Autodesk Fusion 360 part; units mm, degrees
note: some values were not read from the file. Set by a fixed rule: which face or edge a step refers to.
(part 5 of 5)
fillet "Fillet1''''''" radius 11.5 1 edges at (7, -47.65, -17.015) on bodies 23 in component "L_F_Wheel_Base"
fillet "Fillet2'''''''" radius 14 1 edges at (16, -47.65, -17.015) on bodies 23 in component "L_F_Wheel_Base"
sketch "Sketch5 (9)" plane through (0, 0, -26.015) normal (0, 0, -1) x (-1, 0, 0) in component "L_F_Wheel_Base"
  arc A0 (-16, -38.3973) -> (-10.1604, -49.7731) centre (-2, -38.3973) ccw
  arc A1 (-5.5, -57.351) -> (-10.1604, -49.7731) centre (-16.8635, -59.1175) ccw
  line L0 (-5.5, -57.351) -> (-5.5, -72.351)
  line L1 (-5.5, -72.351) -> (9.5, -72.351)
  line L2 (9.5, -72.351) -> (9.5, -57.351)
  line L3 (9.5, -57.351) -> (-7, -39.65)
  line L4 (-7, -39.65) -> (-7, -31.65)
  line L5 (-7, -31.65) -> (-16, -31.65)
  line L6 (-16, -31.65) -> (-16, -38.3973)
  line L7 (9.5, -57.351) -> (-5.5, -57.351)
  constraint coincident L2.end L3.start
  constraint coincident A1.start L0.start
extrude "Extrude5''''''''" add sketch "Sketch5 (9)" along normal blind 2 contours L0 L1 L2 L7 bodies 23 in component "L_F_Wheel_Base"
extrude "Extrude6''''''''" cut 1 faces at (0.5, -67.351, -6.015) along direction (0, 0, -1) blind 2 on bodies 23 bodies 23 in component "L_F_Wheel_Base"
sketch "Sketch6 (9)" plane through (0, -26.65, 0) normal (0, 1, 0) x (-1, 0, 0) in component "L_F_Wheel_Base"
  circle A0 centre (-11.5, -4.1) radius 1
  circle A1 centre (-11.5, -29.93) radius 1
  line L0 (-5.5, -29.015) -> (-5.5, -5.015)
  line L1 (-5.5, -5.015) -> (-7.1, -5.015)
  line L2 (-7.1, -5.015) -> (-7.1, -0.5642)
  line L3 (-7.1, -0.5642) -> (-15.9, -0.5642)
  line L4 (-15.9, -0.5642) -> (-15.9, -5.015)
  line L5 (-15.9, -5.015) -> (-17.5, -5.015)
  line L6 (-17.5, -5.015) -> (-17.5, -29.015)
  line L7 (-17.5, -29.015) -> (-15.9, -29.015)
  line L8 (-15.9, -29.015) -> (-15.9, -33.466)
  line L9 (-15.9, -33.466) -> (-7.1, -33.466)
  line L10 (-7.1, -33.466) -> (-7.1, -29.015)
  line L11 (-7.1, -29.015) -> (-5.5, -29.015)
  line L12 (-16, -27.03) -> (-7, -27.03)
  line L13 (-16, -7) -> (-16, -27.03)
  line L14 (-7, -27.03) -> (-7, -7)
  line L15 (-7, -27.03) -> (-16, -27.03)
  line L16 (-16, -27.03) -> (-16, -7)
  line L17 (-16, -7) -> (-7, -7)
  line L18 (-7, -7) -> (-7, -27.03)
  line L19 (-15.91, -7.09) -> (-7.09, -7.09)
  line L20 (-7.09, -7.09) -> (-7.09, -26.94)
  line L21 (-7.09, -26.94) -> (-15.91, -26.94)
  line L22 (-15.91, -26.94) -> (-15.91, -7.09)
  dimension "d553_1" = 0.09
  constraint horizontal L15
  constraint vertical L16
  constraint horizontal L17
  constraint vertical L18
  constraint coincident L13.start L16.end
  constraint coincident L12.end L14.start
extrude "Extrude7'''''" add sketch "Sketch6 (9)" along normal blind 3 contours L19 L20 L21 L22 bodies 23 in component "L_F_Wheel_Base"
sketch "Sketch7 (7)" plane through (0, 0, -8.015) normal (0, 0, 1) x (1, 0, 0) in component "L_F_Wheel_Base"
  arc A0 (10.1604, -49.7731) -> (16, -38.3973) centre (2, -38.3973) ccw
  line L0 (16, -38.3973) -> (16, -31.65)
  line L1 (16, -31.65) -> (7, -31.65)
  line L2 (7, -31.65) -> (7, -39.65)
  line L3 (7, -39.65) -> (-9.5, -57.351)
  line L4 (-9.5, -57.351) -> (-9.5, -72.351)
  line L5 (-9.5, -72.351) -> (5.5, -72.351)
  line L6 (5.5, -72.351) -> (5.5, -57.351)
  arc A1 (10.1604, -49.7731) -> (5.5, -57.351) centre (16.8635, -59.1175) ccw
  line L7 (-9.5, -57.351) -> (5.5, -57.351)
  circle A2 centre (-2, -64.851) radius 2
  line L8 (-2, -64.851) -> (-6.572, -64.851) construction
  line L9 (-2, -64.851) -> (2.572, -64.851) construction
  circle A3 centre (-6.572, -64.851) radius 0.75
  circle A4 centre (2.572, -64.851) radius 0.75
  dimension "d556_1" = 4
  dimension "d557_1" = 4.572
  dimension "d558_1" = 4.572
  dimension "d559_1" = 1.5
  dimension "d560_1" = 1.5
  constraint coincident L3.end L4.start
  constraint coincident L6.end A1.end
  constraint coincident A2.centre L8.start
  constraint horizontal L8
  constraint parallel L8 L9
  constraint coincident L8.end A3.centre
  constraint coincident L9.end A4.centre
  measures "d556_1" diameter of A2
  measures "d557_1" distance of A2.centre L8.end
  measures "d558_1" distance of A2.centre L9.end
  measures "d559_1" diameter of A3
  measures "d560_1" diameter of A4
extrude "Extrude8'''''" cut sketch "Sketch7 (7)" against normal blind 20 contours A2 | A3 | A4 bodies 23 in component "L_F_Wheel_Base"
sketch "Sketch8 (4)" plane through (0, 0, -28.015) normal (0, 0, -1) x (-1, 0, 0) in component "L_F_Wheel_Base"
  circle A0 centre (2, -64.851) radius 2
  circle A1 centre (6.572, -64.851) radius 0.75
  circle A2 centre (-2.572, -64.851) radius 0.75
  line L0 (9.5, -57.351) -> (-5.5, -57.351)
  line L1 (-5.5, -57.351) -> (-5.5, -72.351)
  line L2 (-5.5, -72.351) -> (9.5, -72.351)
  line L3 (9.5, -72.351) -> (9.5, -57.351)
  line L4 (8.1, -69.951) -> (-4.1, -69.951)
  line L5 (-4.1, -69.951) -> (-4.1, -59.751)
  line L6 (-4.1, -59.751) -> (8.1, -59.751)
  line L7 (8.1, -59.751) -> (8.1, -69.951)
  line L8 (8.1, -69.951) -> (-4.1, -59.751) construction
  line L9 (-4.1, -69.951) -> (8.1, -59.751) construction
  point P0 (2, -64.851)
  dimension "d563_1" = 12.2
  dimension "d564_1" = 10.2
  constraint horizontal L4
  constraint perpendicular L4 L5
  constraint parallel L4 L6
  constraint parallel L5 L7
  constraint coincident L8 P0
  constraint coincident L9 P0
  constraint coincident P0 A0.centre
  measures "d563_1" distance of L5.end L6.end
  measures "d564_1" distance of L4.end L5.end
extrude "Extrude9''''" cut sketch "Sketch8 (4)" against normal blind 18.841 contours L4 L5 L6 L7 bodies 23 in component "L_F_Wheel_Base"
extrude "Extrude10''" add 1 faces at (0.0333, -59.751, -21.7347) along direction (0, -1, 0) blind 10.2 on bodies 23 bodies 23 in component "L_F_Wheel_Base"
extrude "Extrude11''" cut 3 faces at (-1.7564, -64.1717, -9.174) (-6.3887, -65.021, -9.174) (2.2775, -64.681, -9.174) along direction (0, 0, -1) blind 18.841 on bodies 23 bodies 23 in component "L_F_Wheel_Base"
sketch "Sketch9 (2)" plane through (0, 0, -8.015) normal (0, 0, 1) x (1, 0, 0) in component "L_F_Wheel_Base"
  circle A0 centre (-2, -64.851) radius 2
  circle A1 centre (-6.572, -64.851) radius 0.75
  circle A2 centre (2.572, -64.851) radius 0.75
  arc A3 (10.1604, -49.7731) -> (16, -38.3973) centre (2, -38.3973) ccw
  line L0 (16, -38.3973) -> (16, -31.65)
  line L1 (16, -31.65) -> (7, -31.65)
  line L2 (7, -31.65) -> (7, -39.65)
  line L3 (7, -39.65) -> (-9.5, -57.351)
  line L4 (-9.5, -57.351) -> (-9.5, -72.351)
  line L5 (-9.5, -72.351) -> (5.5, -72.351)
  line L6 (5.5, -72.351) -> (5.5, -57.351)
  arc A4 (10.1604, -49.7731) -> (5.5, -57.351) centre (16.8635, -59.1175) ccw
  line L7 (-9.5, -57.351) -> (5.5, -57.351)
  constraint coincident L3.end L4.start
  constraint coincident L6.end A4.end
extrude "Extrude12''" add sketch "Sketch9 (2)" along normal blind 2 contours L4 L5 L6 L7 bodies 23 in component "L_F_Wheel_Base"
extrude "Extrude13'''" cut 1 faces at (-2.0498, -70.5158, -28.015) along direction (0, 0, 1) blind 2 on bodies 23 bodies 23 in component "L_F_Wheel_Base"
sketch "Sketch10 (2)" plane through (0, 0, -6.015) normal (0, 0, 1) x (1, 0, 0) in component "L_F_Wheel_Base"
  circle A0 centre (2.572, -64.851) radius 0.75
  circle A1 centre (-2, -64.851) radius 2
  circle A2 centre (-6.572, -64.851) radius 0.75
  line L0 (-9.5, -72.351) -> (5.5, -72.351)
  line L1 (5.5, -72.351) -> (5.5, -57.351)
  line L2 (5.5, -57.351) -> (-9.5, -57.351)
  line L3 (-9.5, -57.351) -> (-9.5, -72.351)
  line L4 (4.1, -69.951) -> (-8.1, -69.951)
  line L5 (-8.1, -69.951) -> (-8.1, -59.751)
  line L6 (-8.1, -59.751) -> (4.1, -59.751)
  line L7 (4.1, -59.751) -> (4.1, -69.951)
  line L8 (4.1, -69.951) -> (-8.1, -59.751) construction
  line L9 (-8.1, -69.951) -> (4.1, -59.751) construction
  point P0 (-2, -64.851)
  dimension "d575" = 12.2
  dimension "d576" = 10.2
  constraint horizontal L4
  constraint perpendicular L4 L5
  constraint parallel L4 L6
  constraint parallel L5 L7
  constraint coincident L8 P0
  constraint coincident L9 P0
  constraint coincident P0 A1.centre
  measures "d575" distance of L5.end L6.end
  measures "d576" distance of L4.end L5.end
extrude "Extrude14''" cut sketch "Sketch10 (2)" against normal blind 18.841 contours L4 L5 L6 L7 bodies 23 in component "L_F_Wheel_Base"
ref_plane "WorkPlane1" through (3.25, -52.0005, 1.985) normal (0, 0, 1) x (-1, 0, 0)
sketch "Sketch7 (1)" plane through (3.25, -52.0005, 1.985) normal (0, 0, 1) x (1, 0, 0)
  circle A0 centre (-5.25, -12.8505) radius 2
  circle A1 centre (-5.25, -12.8505) radius 25
  dimension "d580" = 50
  constraint concentric A0 A1
  measures "d580" diameter of A1
extrude "Extrude2''''''''''''''" add sketch "Sketch7 (1)" along normal blind 10 separate body contours A0 | A1 makes body 24
fillet "Fillet1'''''''" radius 1.5 2 edges at (-25.3082, -73.8914, 11.985) (-25.3082, -73.8914, 1.985) on bodies 24
sketch "Sketch7 (8)" plane through (0, 0, 11.985) normal (0, 0, 1) x (1, 0, 0)
  circle A0 centre (-2, -64.851) radius 23.5
  circle A1 centre (-2, -64.851) radius 1.55
  line L0 (-2, -64.851) -> (-2, -54.851)
  circle A2 centre (-2, -54.851) radius 2.1
  circle A3 centre (-9.0711, -57.7799) radius 2.1
  circle A4 centre (-12, -64.851) radius 2.1
  circle A5 centre (-9.0711, -71.9221) radius 2.1
  circle A6 centre (-2, -74.851) radius 2.1
  circle A7 centre (5.0711, -71.9221) radius 2.1
  circle A8 centre (8, -64.851) radius 2.1
  circle A9 centre (5.0711, -57.7799) radius 2.1
  dimension "d584" = 3.1
  dimension "d585" = 10
  dimension "d586" = 4.2
  dimension "d588" = 360
  constraint concentric A0 A1
  constraint coincident A0.centre A1.centre
  constraint vertical L0
  constraint coincident L0.end A2.centre
  measures "d584" diameter of A1
  measures "d585" distance of A0.centre L0.end
  measures "d586" diameter of A2
extrude "Extrude3''''''''''''" cut sketch "Sketch7 (8)" against normal blind 10 contours A1 | A2 | A3 | A4 | A5 | A6 | A7 | A8 | A9 bodies 24
copy_body "CutPasteBodies1" bodies 24 removing the originals makes body 25 in component "Wheel"
extrude "Extrude9'''''" cut 1 faces at (115.1632, -31.65, -27.6457) along direction (0, 1, 0) blind 3 on bodies 18 bodies 18 in component "R_R_Wheel_Base"
fillet "Fillet4'" radius 1 4 edges at (102.5, -28.65, -28) (112, -28.65, -23.47) (102.5, -28.65, -18.94) (93, -28.65, -23.47) on bodies 18 in component "R_R_Wheel_Base"
extrude "Extrude14'''" cut 1 faces at (115.1632, -31.65, -27.6457) along direction (0, 1, 0) blind 3 on bodies 21 bodies 21 in component "L_R_Wheel_Base"
fillet "Fillet4''" radius 1 4 edges at (102.5, -28.65, -28) (93, -28.65, -23.47) (102.5, -28.65, -18.94) (112, -28.65, -23.47) on bodies 21 in component "L_R_Wheel_Base"
extrude "Extrude10'''" cut 1 faces at (11.5249, -31.65, -26.9876) along direction (0, 1, 0) blind 3 on bodies 22 bodies 22 in component "R_F_Wheel_Base"
fillet "Fillet3'" radius 1 4 edges at (7, -28.65, -17.015) (11.5, -28.65, -26.015) (11.5, -28.65, -8.015) (16, -28.65, -17.015) on bodies 22 in component "R_F_Wheel_Base"
extrude "Extrude15'''" cut 1 faces at (11.5249, -31.65, -26.9876) along direction (0, 1, 0) blind 3 on bodies 23 bodies 23 in component "L_F_Wheel_Base"
fillet "Fillet3''" radius 1 4 edges at (7, -28.65, -17.015) (11.5, -28.65, -26.015) (16, -28.65, -17.015) (11.5, -28.65, -8.015) on bodies 23 in component "L_F_Wheel_Base"
ref_plane "WorkPlane2" through (-2, -64.851, 10.485) normal (0, 0, 1) x (1, 0, 0)
sketch "Sketch1 (14)" plane through (-2, -64.851, 10.485) normal (0, 0, 1) x (1, 0, 0) in component "Wheel"
  circle A0 centre (0, 0) radius 25
  circle A1 centre (0, 0) radius 24.15
  dimension "d604" = 50
  dimension "d605" = -0.85
  constraint coincident A0.centre A1.centre
  measures "d604" diameter of A0
extrude "Extrude1''''''''''''''''" cut sketch "Sketch1 (14)" against normal blind 2 bodies 25 in component "Wheel"
sketch "Sketch7 (9)" plane through (-8, 0, 0) normal (-1, 0, 0) x (0, 0, 1) in component "Ultrasonic_Sensor_Mount"
  line L0 (-33, 43.3) -> (-33, 38.5)
  arc A0 (-45.5, 26) -> (-33, 38.5) centre (-45.5, 38.5) ccw
  line L1 (-45.5, 26) -> (-54.5, 26)
  arc A1 (-67, 38.5) -> (-54.5, 26) centre (-54.5, 38.5) ccw
  line L2 (-67, 38.5) -> (-67, 43.3)
  line L3 (-67, 43.3) -> (-72.85, 43.3)
  line L4 (-72.85, 43.3) -> (-72.85, 22)
  line L5 (-72.85, 22) -> (-58, 22)
  line L6 (-58, 22) -> (-42, 22)
  line L7 (-42, 22) -> (-27.15, 22)
  line L8 (-27.15, 22) -> (-27.15, 43.3)
  line L9 (-27.15, 43.3) -> (-33, 43.3)
  circle A2 centre (-29.65, 40.8) radius 2
  circle A3 centre (-70.35, 24.5) radius 2
  line L10 (-33, 43.3) -> (-27.15, 43.3)
  line L11 (-27.15, 43.3) -> (-27.15, 37.45)
  line L12 (-27.15, 37.45) -> (-33, 37.45)
  line L13 (-33, 37.45) -> (-33, 43.3)
  line L14 (-72.85, 22) -> (-67, 22)
  line L15 (-67, 22) -> (-67, 27.85)
  line L16 (-67, 27.85) -> (-72.85, 27.85)
  line L17 (-72.85, 27.85) -> (-72.85, 22)
  dimension "d608" = 5.85
  dimension "d609" = 5.85
  constraint horizontal L10
  constraint vertical L11
  constraint horizontal L12
  constraint vertical L13
  constraint coincident L0.start L9.end
  constraint horizontal L14
  constraint vertical L15
  constraint horizontal L16
  constraint vertical L17
  constraint coincident L4.end L5.start
  measures "d608" distance of L0.start L12.end
  measures "d609" distance of L4.end L16.end
extrude "Extrude7''''''" add sketch "Sketch7 (9)" along normal blind 2 contours L0 L8 L9 L10 L11 L12 L13 | L4 L5 L14 L15 L16 L17 bodies 10 in component "Ultrasonic_Sensor_Mount"
sketch "Sketch8 (5)" plane through (0, 0, -13.97) normal (0, 0, -1) x (-1, 0, 0) in component "LCD_Mount"
  line L0 (-114.3, 42) -> (-115, 42)
  line L1 (-115, 42) -> (-119, 46)
  line L2 (-119, 46) -> (-119, 1.57)
  line L3 (-119, 1.57) -> (-119, 0)
  line L4 (-119, 0) -> (-114.32, 0)
  line L5 (-114.32, 0) -> (-114.32, 1.57)
  line L6 (-114.32, 1.57) -> (-114.3, 1.57)
  line L7 (-114.3, 1.57) -> (-114.3, 4.57)
  line L8 (-114.3, 4.57) -> (-114.3, 42)
  line L9 (-114.3, 1.57) -> (-119, 1.57)
  line L10 (-119, 1.57) -> (-119, 0)
  line L11 (-119, 0) -> (-114.3, 0)
  line L12 (-114.3, 0) -> (-114.3, 1.57)
  constraint horizontal L9
  constraint vertical L10
  constraint horizontal L11
  constraint vertical L12
  constraint coincident L3.end L4.start
  constraint coincident L6.end L7.start
extrude "Extrude10''''" cut sketch "Sketch8 (5)" against normal blind 0.5 contours L3 L4 L5 L9 L10 L11 bodies 16 in component "LCD_Mount"
sketch "Sketch9 (3)" plane through (0, 0, -3.81) normal (0, 0, 1) x (1, 0, 0) in component "LCD_Mount"
  line L0 (114.32, 1.57) -> (114.32, 0)
  line L1 (114.32, 0) -> (119, 0)
  line L2 (119, 0) -> (119, 1.57)
  line L3 (119, 1.57) -> (119.0032, 1.57)
  line L4 (119.0032, 1.57) -> (119.0032, 54.57)
  line L5 (119.0032, 54.57) -> (114.3, 54.57)
  line L6 (114.3, 54.57) -> (114.3, 4.57)
  line L7 (114.3, 4.57) -> (98, 4.57)
  line L8 (98, 4.57) -> (98, 1.57)
  line L9 (98, 1.57) -> (114.32, 1.57)
  line L10 (114.32, 1.57) -> (119, 1.57)
  line L11 (119, 1.57) -> (119, 0)
  line L12 (119, 0) -> (114.32, 0)
  line L13 (114.32, 0) -> (114.32, 1.57)
  constraint horizontal L10
  constraint vertical L11
  constraint horizontal L12
  constraint vertical L13
  constraint coincident L1.end L2.start
  constraint coincident L0.start L9.end
extrude "Extrude11'''" cut sketch "Sketch9 (3)" against normal blind 0.5 contours L0 L1 L2 L10 L11 L12 L13 bodies 16 in component "LCD_Mount"
extrude "Extrude2'''''''''''''''" cut 1 faces at (4.6901, -88.5809, 8.485) along direction (0, 0, -1) blind 5 on bodies 25 bodies 25 in component "Wheel"
